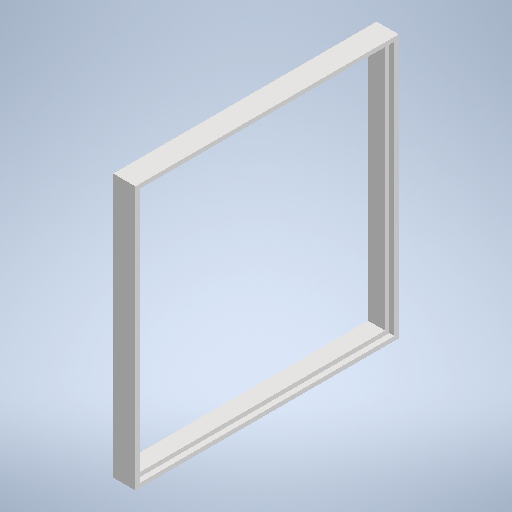
# Autodesk Inventor part: rebord1515
Saved by Autodesk Inventor 2025.2 (Build 292293000, 293)
## iProperties
Created: 2025-02-22
Part Number: rebord1515
Material: Générique
Document SubType Name: Modeling
Designer: antoi
Density: 1 g/cm^3
Appearance: Par défaut
Author: antoi
Autodesk Inventor part; units mm, degrees
ref_plane "YZ Plane" through (0, 0, 0) normal (1, 0, 0) x (0, 1, 0)
ref_plane "XZ Plane" through (0, 0, 0) normal (0, 1, 0) x (-1, 0, 0)
ref_plane "XY Plane" through (0, 0, 0) normal (0, 0, 1) x (1, 0, 0)
sketch "Esquisse1" plane through (0, 0, 0) normal (1, 0, 0) x (0, 1, 0)
  line L0 (0, 0) -> (155, 0)
  line L1 (155, 0) -> (155, -155)
  line L2 (155, -155) -> (0, -155)
  line L3 (0, -155) -> (0, 0)
  line L4 (5, -5) -> (150, -5)
  line L5 (150, -5) -> (150, -150)
  line L6 (150, -150) -> (5, -150)
  line L7 (5, -150) -> (5, -5)
  dimension "d0" = 155
  dimension "d1" = 155
  dimension "d2" = 145
  dimension "d3" = 145
  constraints: 16 end point, 4 parallel, 2 horizontal, 2 perpendicular
  measures "d0" distance of L1.end L2.end
  measures "d1" distance of L0.end L1.end
  measures "d2" distance of L5.end L6.end
  measures "d3" distance of L4.end L5.end
extrude "Extrusion1" add sketch "Esquisse1" along normal blind 13
sketch "Esquisse2" plane through (13, 0, 0) normal (1, 0, 0) x (0, 0, -1)
  line L0 (2.5, 2.5) -> (152.5, 2.5)
  line L1 (152.5, 2.5) -> (152.5, 152.5)
  line L2 (152.5, 152.5) -> (2.5, 152.5)
  line L3 (2.5, 152.5) -> (2.5, 2.5)
  line L4 (150, 5) -> (5, 5) projected
  line L5 (5, 5) -> (150, 5)
  line L6 (150, 5) -> (150, 150)
  line L7 (150, 150) -> (5, 150)
  line L8 (5, 150) -> (5, 5)
  point P0 (0, 0)
  point P1 (155, 155)
  dimension "d7" = 150
  dimension "d8" = 150
  constraints: 16 end point, 4 parallel, 2 horizontal, 2 perpendicular
  measures "d7" distance of L2.end L1.end
  measures "d8" distance of L1.end L0.end
extrude "Extrusion2" cut sketch "Esquisse2" against normal blind 3
